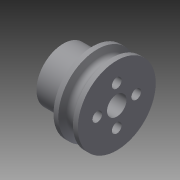
# Autodesk Inventor part: motor_trinse
Saved by Autodesk Inventor 2015 (Build 190159000, 159)
## iProperties
Created: 2015-03-04
Part Number: motor_trinse
Material: Generic
Document SubType Name: Modeling
Designer: Simen
Density: 1 g/cm^3
Appearance: Default
Author: Simen
Autodesk Inventor part; units mm, degrees
ref_plane "YZ Plane" through (0, 0, 0) normal (1, 0, 0) x (0, 1, 0)
ref_plane "XZ Plane" through (0, 0, 0) normal (0, 1, 0) x (-1, 0, 0)
ref_plane "XY Plane" through (0, 0, 0) normal (0, 0, 1) x (1, 0, 0)
sketch "Sketch1" plane through (0, 0, 0) normal (0, 0, 1) x (1, 0, 0)
  line L0 (4.9734, -6.5186) -> (-5.17, -6.5186) construction
  line L1 (-5.1132, 9.4814) -> (-5.1132, 4.4814)
  line L2 (-5.1132, -2.5186) -> (4.8868, -2.5186)
  line L3 (4.8868, 9.4814) -> (2.8868, 9.4814)
  line L4 (2.8868, 9.4814) -> (1.5056, 7.4814)
  arc A0 (-1.9585, 7.4814) -> (1.5056, 7.4814) centre (-0.2265, 8.4814) ccw
  line L5 (-1.9585, 7.4814) -> (-3.1132, 9.4814)
  line L6 (-3.1132, 9.4814) -> (-5.1132, 9.4814)
  line L7 (4.8868, 9.4814) -> (4.8868, -2.5186)
  line L8 (-5.1132, 4.4814) -> (-17.1132, 4.4814)
  line L9 (-17.1132, 4.4814) -> (-17.1132, -2.5186)
  line L10 (-17.1132, -2.5186) -> (-5.1132, -2.5186)
  dimension "d28" = 2
  dimension "d29" = 120
  dimension "d30" = 12
  dimension "d31" = 10
  dimension "d32" = 4
  dimension "d33" = 2
  dimension "d34" = 2
  dimension "d35" = 2
  dimension "d36" = 2
  dimension "d45" = 12
  dimension "d48" = 11
  constraints: 22 end point, 4 perpendicular, 2 collinear, 2 horizontal, 2 parallel, 2 point on circle, 1 centre point, 1 tangent
  measures "d28" radius of A0
  measures "d30" distance of L3.start L2.end
  measures "d31" distance of L2.start L2.end
  measures "d32" distance from line of L0 L2.end
  measures "d33" distance of L3.start L3.end
  measures "d34" distance of L5.end L1.start
  measures "d35" vertical distance of L5.start L5.end
  measures "d36" vertical distance of L3.end L4.end
  measures "d45" distance of L2.start L9.end
  measures "d48" distance between parallel lines of L0 L8
revolve "Revolution1" add sketch "Sketch1" angle 360 about axis through (4.9734, -6.5186, 0) along (-1, 0, 0)
sketch "Sketch3" plane through (4.8868, -6.5186, 0) normal (1, 0, 0) x (0, 0, -1)
  circle A0 centre (0, 0) radius 4 projected
  line L0 (0, 0) -> (-8, 0) construction
  point P0 (0, 6.5186)
  point P1 (0, -8)
  point P2 (8, 0)
  point P3 (0, 8)
  dimension "d49" = 8
  dimension "d52" = 360
  constraints: 2 end point, 1 coincident, 1 horizontal, 5 other
  measures "d49" distance of L0.start L0.end
hole "Hole2" at (4.8868, -6.5186, 0) at (4.8868, -6.5186, 8) at (4.8868, -14.5186, 0) at (4.8868, -6.5186, -8) at (4.8868, 1.4814, 0) direction (-1, 0, 0) diameter 2.4 end through all counterbore diameter 4 counterbore depth 18
body "Solid1"
